增高架-2 (Autodesk Fusion 360 design; units mm, degrees)
part number: 2026-05-03-11-57-41-688
Autodesk Fusion 360 part; units mm, degrees
(part 1 of 12)
sketch "草图2" plane through (0, 0, 0) normal (0, 0, 1) x (1, 0, 0)
  line L0 (70.0002, -75) -> (70, 65) construction
  line L1 (60, 75) -> (-60, 75) construction
  line L2 (-70, 65) -> (-69.9998, -75) construction
  line L3 (-60, 75) -> (60, 75) construction
  line L4 (70, 85) -> (70, 165) construction
  line L5 (70, 165) -> (-70, 165) construction
  line L6 (-70, 165) -> (-70, 85) construction
  arc A0 (-70, 85) -> (-60, 75) centre (-60, 85) ccw construction
  arc A1 (-60, 75) -> (-70, 65) centre (-60, 65) ccw construction
  arc A2 (60, 75) -> (70, 85) centre (60, 85) ccw construction
  arc A3 (70, 65) -> (60, 75) centre (60, 65) ccw construction
  line L7 (-71.4998, -74.9987) -> (-68.4998, -74.9988)
  line L8 (68.5002, -74.9988) -> (71.5002, -74.9987)
  line L9 (68.5002, -74.9988) -> (68.5, 65)
  line L10 (71.5002, -74.9987) -> (71.5, 65)
  line L11 (60, 73.5) -> (-60, 73.5)
  line L12 (60, 76.5) -> (-60, 76.5)
  line L13 (-68.5, 65) -> (-68.4998, -74.9988)
  line L14 (-71.5, 65) -> (-71.4998, -74.9987)
  line L15 (68.5, 85.0003) -> (68.4999, 155)
  line L16 (71.5, 85.0232) -> (71.4999, 161.5)
  line L17 (59.9999, 163.5) -> (-60.0001, 163.5)
  line L18 (66.4999, 166.5) -> (-66.5001, 166.5)
  line L19 (-68.5001, 155) -> (-68.5, 85.0003)
  line L20 (-71.5001, 161.5) -> (-71.5, 85.0009)
  arc A4 (-68.5, 85.0003) -> (-60, 76.5) centre (-60, 85) ccw
  arc A5 (-60, 73.5) -> (-68.5, 65) centre (-60, 65) ccw
  arc A6 (60, 76.5) -> (68.5, 85.0003) centre (60, 85) ccw
  arc A7 (68.5, 65) -> (60, 73.5) centre (60, 65) ccw
  line L21 (-70, 65) -> (-70, 85) construction
  line L22 (70, 65) -> (70, 85) construction
  arc A8 (-71.5, 85.0009) -> (-71.5, 84.9991) centre (-60, 85) ccw
  arc A9 (71.5, 84.9769) -> (71.5, 85.0232) centre (60, 85) ccw
  line L23 (-71.5, 85.0009) -> (-71.5, 65)
  line L24 (71.5, 85.0232) -> (71.5, 65)
  arc A10 (-60.0001, 163.5) -> (-68.5001, 155) centre (-60.0001, 155) ccw
  arc A11 (-66.5001, 166.5) -> (-71.5001, 161.5) centre (-66.5001, 161.5) ccw
  arc A12 (68.4999, 155) -> (59.9999, 163.5) centre (59.9999, 155) ccw
  arc A13 (71.4999, 161.5) -> (66.4999, 166.5) centre (66.4999, 161.5) ccw
  dimension "d1" = 140
  dimension "d3" = 90
  dimension "d4" = 10
  dimension "d5" = 10
  dimension "d6" = 10
  dimension "d7" = 10
  dimension "d13" = 1.5
  dimension "d14" = 1.5
  dimension "d15" = 1.5
  dimension "d18" = 8.5
  dimension "d21" = 8.5
  dimension "d23" = 1.5
  dimension "d24" = 1.5
  dimension "d25" = 1.5
  dimension "d26" = 1.5
  dimension "d27" = 8.5
  dimension "d28" = 8.5
  dimension "d29" = 11.5
  dimension "d31" = 11.5
  dimension "d40" = 8.5
  dimension "d41" = 5
  dimension "d42" = 8.5
  dimension "d43" = 5
  constraint parallel L0 L2
  constraint perpendicular L3 L4
  constraint parallel L3 L5
  constraint parallel L4 L6
  constraint tangent L6 A0
  constraint tangent L3 A0
  constraint coincident L3 L1.end
  constraint tangent L3 A1
  constraint tangent L2 A1
  constraint tangent L4 A2
  constraint tangent L3 A2
  constraint tangent L1 A3
  constraint tangent L0 A3
  constraint coincident L7.start L14.end
  constraint coincident L7.end L13.end
  constraint coincident L8.start L9.start
  constraint coincident L8.end L10.start
  constraint coincident L9.end A7.start
  constraint coincident L11.start A7.end
  constraint coincident L11.end A5.start
  constraint coincident L12.start A6.start
  constraint coincident L12.end A4.end
  constraint coincident L13.start A5.end
  constraint coincident L15.start A6.end
  constraint coincident L19.end A4.start
  constraint parallel L0 L9
  constraint parallel L0 L10
  constraint parallel L1 L11
  constraint parallel L1 L12
  constraint parallel L2 L13
  constraint parallel L2 L14
  constraint parallel L0 L15
  constraint parallel L0 L16
  constraint parallel L5 L17
  constraint parallel L5 L18
  constraint parallel L2 L19
  constraint parallel L2 L20
  constraint concentric A0 A4
  constraint concentric A1 A5
  constraint concentric A2 A6
  constraint concentric A3 A7
  constraint coincident L2.start A1.end
  constraint coincident L6.end A0.start
  constraint coincident L0.end A3.start
  constraint coincident L4.start A2.end
  constraint coincident L16.start A9.end
  constraint coincident L20.end A8.start
  constraint concentric A0 A8
  constraint concentric A2 A9
  constraint coincident L23 A8.end
  constraint coincident L24 A9.start
  constraint tangent L17 A10
  constraint tangent L19 A10
  constraint tangent L20 A11
  constraint tangent L18 A11
  constraint tangent L17 A12
  constraint tangent L15 A12
  constraint tangent L16 A13
  constraint tangent L18 A13
  measures "d1" distance of L0 L2
  measures "d3" distance of L1 L5
  measures "d4" radius of A0
  measures "d5" radius of A1
  measures "d6" radius of A2
  measures "d7" radius of A3
  measures "d13" distance of L1 L11
  measures "d14" distance of L1 L12
  measures "d15" distance of L5 L17
  measures "d18" radius of A4
  measures "d21" radius of A6
  measures "d23" distance of L0 L9
  measures "d24" distance of L0 L10
  measures "d25" distance of L2 L13
  measures "d26" distance of L2 L14
  measures "d27" radius of A5
  measures "d28" radius of A7
  measures "d29" radius of A8
  measures "d31" radius of A9
  measures "d40" radius of A10
  measures "d41" radius of A11
  measures "d42" radius of A12
  measures "d43" radius of A13
extrude "拉伸1" add sketch "草图2" along normal blind 250 contours L7 L13 L14 A5 A8 L23 | L12 L19 A4 A8 | L8 L9 L10 L11 L12 L15 L16 L17 L18 L19 L20 A6 A7 A8 A9 L24 A10 A11 A12 A13 picked at (-59.4355, 74.5418)
sketch "草图18" plane through (0, 166.5, 0) normal (0, 1, 0) x (-1, 0, 0)
  line L0 (-66.4999, 0) -> (66.5001, 0)
  line L1 (66.5001, 0) -> (66.5001, 250)
  line L2 (66.5001, 250) -> (-66.4999, 250)
  line L3 (-66.4999, 250) -> (-66.4999, 0)
  line L4 (-56.4999, 15) -> (-60.83, 12.5)
  line L5 (-60.83, 12.5) -> (-60.83, 7.5)
  line L6 (-60.83, 7.5) -> (-56.4999, 5)
  line L7 (-56.4999, 5) -> (-52.1698, 7.5)
  line L8 (-52.1698, 7.5) -> (-52.1698, 12.5)
  line L9 (-52.1698, 12.5) -> (-56.4999, 15)
  line L10 (-45.8396, 15) -> (-50.1698, 12.5)
  line L11 (-50.1698, 12.5) -> (-50.1698, 7.5)
  line L12 (-50.1698, 7.5) -> (-45.8396, 5)
  line L13 (-45.8396, 5) -> (-41.5095, 7.5)
  line L14 (-41.5095, 7.5) -> (-41.5095, 12.5)
  line L15 (-41.5095, 12.5) -> (-45.8396, 15)
  line L16 (-35.1794, 15) -> (-39.5095, 12.5)
  line L17 (-39.5095, 12.5) -> (-39.5095, 7.5)
  line L18 (-39.5095, 7.5) -> (-35.1794, 5)
  line L19 (-35.1794, 5) -> (-30.8493, 7.5)
  line L20 (-30.8493, 7.5) -> (-30.8493, 12.5)
  line L21 (-30.8493, 12.5) -> (-35.1794, 15)
  line L22 (-24.5191, 15) -> (-28.8493, 12.5)
  line L23 (-28.8493, 12.5) -> (-28.8493, 7.5)
  line L24 (-28.8493, 7.5) -> (-24.5191, 5)
  line L25 (-24.5191, 5) -> (-20.189, 7.5)
  line L26 (-20.189, 7.5) -> (-20.189, 12.5)
  line L27 (-20.189, 12.5) -> (-24.5191, 15)
  line L28 (-13.8589, 15) -> (-18.189, 12.5)
  line L29 (-18.189, 12.5) -> (-18.189, 7.5)
  line L30 (-18.189, 7.5) -> (-13.8589, 5)
  line L31 (-13.8589, 5) -> (-9.5287, 7.5)
  line L32 (-9.5287, 7.5) -> (-9.5287, 12.5)
  line L33 (-9.5287, 12.5) -> (-13.8589, 15)
  line L34 (-3.1986, 15) -> (-7.5287, 12.5)
  line L35 (-7.5287, 12.5) -> (-7.5287, 7.5)
  line L36 (-7.5287, 7.5) -> (-3.1986, 5)
  line L37 (-3.1986, 5) -> (1.1315, 7.5)
  line L38 (1.1315, 7.5) -> (1.1315, 12.5)
  line L39 (1.1315, 12.5) -> (-3.1986, 15)
  line L40 (7.4616, 15) -> (3.1315, 12.5)
  line L41 (3.1315, 12.5) -> (3.1315, 7.5)
  line L42 (3.1315, 7.5) -> (7.4616, 5)
  line L43 (7.4616, 5) -> (11.7918, 7.5)
  line L44 (11.7918, 7.5) -> (11.7918, 12.5)
  line L45 (11.7918, 12.5) -> (7.4616, 15)
  line L46 (18.1219, 15) -> (13.7918, 12.5)
  line L47 (13.7918, 12.5) -> (13.7918, 7.5)
  line L48 (13.7918, 7.5) -> (18.1219, 5)
  line L49 (18.1219, 5) -> (22.452, 7.5)
  line L50 (22.452, 7.5) -> (22.452, 12.5)
  line L51 (22.452, 12.5) -> (18.1219, 15)
  line L52 (28.7821, 15) -> (24.452, 12.5)
  line L53 (24.452, 12.5) -> (24.452, 7.5)
  line L54 (24.452, 7.5) -> (28.7821, 5)
  line L55 (28.7821, 5) -> (33.1123, 7.5)
  line L56 (33.1123, 7.5) -> (33.1123, 12.5)
  line L57 (33.1123, 12.5) -> (28.7821, 15)
  line L58 (39.4424, 15) -> (35.1123, 12.5)
  line L59 (35.1123, 12.5) -> (35.1123, 7.5)
  line L60 (35.1123, 7.5) -> (39.4424, 5)
  line L61 (39.4424, 5) -> (43.7725, 7.5)
  line L62 (43.7725, 7.5) -> (43.7725, 12.5)
  line L63 (43.7725, 12.5) -> (39.4424, 15)
  line L64 (50.1027, 15) -> (45.7725, 12.5)
  line L65 (45.7725, 12.5) -> (45.7725, 7.5)
  line L66 (45.7725, 7.5) -> (50.1027, 5)
  line L67 (50.1027, 5) -> (54.4328, 7.5)
  line L68 (54.4328, 7.5) -> (54.4328, 12.5)
  line L69 (54.4328, 12.5) -> (50.1027, 15)
  line L70 (-51.1698, 24.2321) -> (-55.4999, 21.7321)
  line L71 (-55.4999, 21.7321) -> (-55.4999, 16.7321)
  line L72 (-55.4999, 16.7321) -> (-51.1698, 14.2321)
  line L73 (-51.1698, 14.2321) -> (-46.8396, 16.7321)
  line L74 (-46.8396, 16.7321) -> (-46.8396, 21.7321)
  line L75 (-46.8396, 21.7321) -> (-51.1698, 24.2321)
  line L76 (-40.5095, 24.2321) -> (-44.8396, 21.7321)
  line L77 (-44.8396, 21.7321) -> (-44.8396, 16.7321)
  line L78 (-44.8396, 16.7321) -> (-40.5095, 14.2321)
  line L79 (-40.5095, 14.2321) -> (-36.1794, 16.7321)
  line L80 (-36.1794, 16.7321) -> (-36.1794, 21.7321)
  line L81 (-36.1794, 21.7321) -> (-40.5095, 24.2321)
  line L82 (-29.8493, 24.2321) -> (-34.1794, 21.7321)
  line L83 (-34.1794, 21.7321) -> (-34.1794, 16.7321)
  line L84 (-34.1794, 16.7321) -> (-29.8493, 14.2321)
  line L85 (-29.8493, 14.2321) -> (-25.5191, 16.7321)
  line L86 (-25.5191, 16.7321) -> (-25.5191, 21.7321)
  line L87 (-25.5191, 21.7321) -> (-29.8493, 24.2321)
  line L88 (-19.189, 24.2321) -> (-23.5191, 21.7321)
  line L89 (-23.5191, 21.7321) -> (-23.5191, 16.7321)
  line L90 (-23.5191, 16.7321) -> (-19.189, 14.2321)
  line L91 (-19.189, 14.2321) -> (-14.8589, 16.7321)
  line L92 (-14.8589, 16.7321) -> (-14.8589, 21.7321)
  line L93 (-14.8589, 21.7321) -> (-19.189, 24.2321)
  line L94 (-8.5287, 24.2321) -> (-12.8589, 21.7321)
  line L95 (-12.8589, 21.7321) -> (-12.8589, 16.7321)
  line L96 (-12.8589, 16.7321) -> (-8.5287, 14.2321)
  line L97 (-8.5287, 14.2321) -> (-4.1986, 16.7321)
  line L98 (-4.1986, 16.7321) -> (-4.1986, 21.7321)
  line L99 (-4.1986, 21.7321) -> (-8.5287, 24.2321)
  line L100 (2.1315, 24.2321) -> (-2.1986, 21.7321)
  line L101 (-2.1986, 21.7321) -> (-2.1986, 16.7321)
  line L102 (-2.1986, 16.7321) -> (2.1315, 14.2321)
  line L103 (2.1315, 14.2321) -> (6.4616, 16.7321)
  line L104 (6.4616, 16.7321) -> (6.4616, 21.7321)
  line L105 (6.4616, 21.7321) -> (2.1315, 24.2321)
  line L106 (12.7918, 24.2321) -> (8.4616, 21.7321)
  line L107 (8.4616, 21.7321) -> (8.4616, 16.7321)
  line L108 (8.4616, 16.7321) -> (12.7918, 14.2321)
  line L109 (12.7918, 14.2321) -> (17.1219, 16.7321)
  line L110 (17.1219, 16.7321) -> (17.1219, 21.7321)
  line L111 (17.1219, 21.7321) -> (12.7918, 24.2321)
  line L112 (23.452, 24.2321) -> (19.1219, 21.7321)
  line L113 (19.1219, 21.7321) -> (19.1219, 16.7321)
  line L114 (19.1219, 16.7321) -> (23.452, 14.2321)
  line L115 (23.452, 14.2321) -> (27.7821, 16.7321)
  line L116 (27.7821, 16.7321) -> (27.7821, 21.7321)
  line L117 (27.7821, 21.7321) -> (23.452, 24.2321)
  line L118 (34.1123, 24.2321) -> (29.7821, 21.7321)
  line L119 (29.7821, 21.7321) -> (29.7821, 16.7321)
  line L120 (29.7821, 16.7321) -> (34.1123, 14.2321)
  line L121 (34.1123, 14.2321) -> (38.4424, 16.7321)
  line L122 (38.4424, 16.7321) -> (38.4424, 21.7321)
  line L123 (38.4424, 21.7321) -> (34.1123, 24.2321)
  line L124 (44.7725, 24.2321) -> (40.4424, 21.7321)
  line L125 (40.4424, 21.7321) -> (40.4424, 16.7321)
  line L126 (40.4424, 16.7321) -> (44.7725, 14.2321)
  line L127 (44.7725, 14.2321) -> (49.1027, 16.7321)
  line L128 (49.1027, 16.7321) -> (49.1027, 21.7321)
  line L129 (49.1027, 21.7321) -> (44.7725, 24.2321)
  line L130 (55.4328, 24.2321) -> (51.1027, 21.7321)
  line L131 (51.1027, 21.7321) -> (51.1027, 16.7321)
  line L132 (51.1027, 16.7321) -> (55.4328, 14.2321)
  line L133 (55.4328, 14.2321) -> (59.7629, 16.7321)
  line L134 (59.7629, 16.7321) -> (59.7629, 21.7321)
  line L135 (59.7629, 21.7321) -> (55.4328, 24.2321)
  line L136 (-56.4999, 33.4641) -> (-60.83, 30.9641)
  line L137 (-60.83, 30.9641) -> (-60.83, 25.9641)
  line L138 (-60.83, 25.9641) -> (-56.4999, 23.4641)
  line L139 (-56.4999, 23.4641) -> (-52.1698, 25.9641)
  line L140 (-52.1698, 25.9641) -> (-52.1698, 30.9641)
  line L141 (-52.1698, 30.9641) -> (-56.4999, 33.4641)
  line L142 (-45.8396, 33.4641) -> (-50.1698, 30.9641)
  line L143 (-50.1698, 30.9641) -> (-50.1698, 25.9641)
  line L144 (-50.1698, 25.9641) -> (-45.8396, 23.4641)
  line L145 (-45.8396, 23.4641) -> (-41.5095, 25.9641)
  line L146 (-41.5095, 25.9641) -> (-41.5095, 30.9641)
  line L147 (-41.5095, 30.9641) -> (-45.8396, 33.4641)
  line L148 (-35.1794, 33.4641) -> (-39.5095, 30.9641)
  line L149 (-39.5095, 30.9641) -> (-39.5095, 25.9641)
  line L150 (-39.5095, 25.9641) -> (-35.1794, 23.4641)
  line L151 (-35.1794, 23.4641) -> (-30.8493, 25.9641)
  line L152 (-30.8493, 25.9641) -> (-30.8493, 30.9641)
  line L153 (-30.8493, 30.9641) -> (-35.1794, 33.4641)
  line L154 (-24.5191, 33.4641) -> (-28.8493, 30.9641)
  line L155 (-28.8493, 30.9641) -> (-28.8493, 25.9641)
  line L156 (-28.8493, 25.9641) -> (-24.5191, 23.4641)
  line L157 (-24.5191, 23.4641) -> (-20.189, 25.9641)
  line L158 (-20.189, 25.9641) -> (-20.189, 30.9641)
  line L159 (-20.189, 30.9641) -> (-24.5191, 33.4641)
  line L160 (-13.8589, 33.4641) -> (-18.189, 30.9641)
  line L161 (-18.189, 30.9641) -> (-18.189, 25.9641)
  line L162 (-18.189, 25.9641) -> (-13.8589, 23.4641)
  line L163 (-13.8589, 23.4641) -> (-9.5287, 25.9641)
  line L164 (-9.5287, 25.9641) -> (-9.5287, 30.9641)
  line L165 (-9.5287, 30.9641) -> (-13.8589, 33.4641)
  line L166 (-3.1986, 33.4641) -> (-7.5287, 30.9641)
  line L167 (-7.5287, 30.9641) -> (-7.5287, 25.9641)
  line L168 (-7.5287, 25.9641) -> (-3.1986, 23.4641)
  line L169 (-3.1986, 23.4641) -> (1.1315, 25.9641)
  line L170 (1.1315, 25.9641) -> (1.1315, 30.9641)
  line L171 (1.1315, 30.9641) -> (-3.1986, 33.4641)
  line L172 (7.4616, 33.4641) -> (3.1315, 30.9641)
  line L173 (3.1315, 30.9641) -> (3.1315, 25.9641)
  line L174 (3.1315, 25.9641) -> (7.4616, 23.4641)
  line L175 (7.4616, 23.4641) -> (11.7918, 25.9641)
  line L176 (11.7918, 25.9641) -> (11.7918, 30.9641)
  line L177 (11.7918, 30.9641) -> (7.4616, 33.4641)
  line L178 (18.1219, 33.4641) -> (13.7918, 30.9641)
  line L179 (13.7918, 30.9641) -> (13.7918, 25.9641)
  line L180 (13.7918, 25.9641) -> (18.1219, 23.4641)
  line L181 (18.1219, 23.4641) -> (22.452, 25.9641)
  line L182 (22.452, 25.9641) -> (22.452, 30.9641)
  line L183 (22.452, 30.9641) -> (18.1219, 33.4641)
  line L184 (28.7821, 33.4641) -> (24.452, 30.9641)
  line L185 (24.452, 30.9641) -> (24.452, 25.9641)
  line L186 (24.452, 25.9641) -> (28.7821, 23.4641)
  line L187 (28.7821, 23.4641) -> (33.1123, 25.9641)
  line L188 (33.1123, 25.9641) -> (33.1123, 30.9641)
  line L189 (33.1123, 30.9641) -> (28.7821, 33.4641)
  line L190 (39.4424, 33.4641) -> (35.1123, 30.9641)
  line L191 (35.1123, 30.9641) -> (35.1123, 25.9641)
  line L192 (35.1123, 25.9641) -> (39.4424, 23.4641)
  line L193 (39.4424, 23.4641) -> (43.7725, 25.9641)
  line L194 (43.7725, 25.9641) -> (43.7725, 30.9641)
  line L195 (43.7725, 30.9641) -> (39.4424, 33.4641)
  line L196 (50.1027, 33.4641) -> (45.7725, 30.9641)
  line L197 (45.7725, 30.9641) -> (45.7725, 25.9641)
  line L198 (45.7725, 25.9641) -> (50.1027, 23.4641)
  line L199 (50.1027, 23.4641) -> (54.4328, 25.9641)
  line L200 (54.4328, 25.9641) -> (54.4328, 30.9641)
  line L201 (54.4328, 30.9641) -> (50.1027, 33.4641)
  line L202 (-51.1698, 42.6962) -> (-55.4999, 40.1962)
  line L203 (-55.4999, 40.1962) -> (-55.4999, 35.1962)
  line L204 (-55.4999, 35.1962) -> (-51.1698, 32.6962)
  line L205 (-51.1698, 32.6962) -> (-46.8396, 35.1962)
  line L206 (-46.8396, 35.1962) -> (-46.8396, 40.1962)
  line L207 (-46.8396, 40.1962) -> (-51.1698, 42.6962)
  line L208 (-40.5095, 42.6962) -> (-44.8396, 40.1962)
  line L209 (-44.8396, 40.1962) -> (-44.8396, 35.1962)
  line L210 (-44.8396, 35.1962) -> (-40.5095, 32.6962)
  line L211 (-40.5095, 32.6962) -> (-36.1794, 35.1962)
  line L212 (-36.1794, 35.1962) -> (-36.1794, 40.1962)
  line L213 (-36.1794, 40.1962) -> (-40.5095, 42.6962)
  line L214 (-29.8493, 42.6962) -> (-34.1794, 40.1962)
  line L215 (-34.1794, 40.1962) -> (-34.1794, 35.1962)
  line L216 (-34.1794, 35.1962) -> (-29.8493, 32.6962)
  line L217 (-29.8493, 32.6962) -> (-25.5191, 35.1962)
  line L218 (-25.5191, 35.1962) -> (-25.5191, 40.1962)
  line L219 (-25.5191, 40.1962) -> (-29.8493, 42.6962)
  line L220 (-19.189, 42.6962) -> (-23.5191, 40.1962)
  line L221 (-23.5191, 40.1962) -> (-23.5191, 35.1962)
  line L222 (-23.5191, 35.1962) -> (-19.189, 32.6962)
  line L223 (-19.189, 32.6962) -> (-14.8589, 35.1962)
  line L224 (-14.8589, 35.1962) -> (-14.8589, 40.1962)
  line L225 (-14.8589, 40.1962) -> (-19.189, 42.6962)
  line L226 (-8.5287, 42.6962) -> (-12.8589, 40.1962)
  line L227 (-12.8589, 40.1962) -> (-12.8589, 35.1962)
  line L228 (-12.8589, 35.1962) -> (-8.5287, 32.6962)
  line L229 (-8.5287, 32.6962) -> (-4.1986, 35.1962)
  line L230 (-4.1986, 35.1962) -> (-4.1986, 40.1962)
  line L231 (-4.1986, 40.1962) -> (-8.5287, 42.6962)
  line L232 (2.1315, 42.6962) -> (-2.1986, 40.1962)
  line L233 (-2.1986, 40.1962) -> (-2.1986, 35.1962)
  line L234 (-2.1986, 35.1962) -> (2.1315, 32.6962)
  line L235 (2.1315, 32.6962) -> (6.4616, 35.1962)
  line L236 (6.4616, 35.1962) -> (6.4616, 40.1962)
  line L237 (6.4616, 40.1962) -> (2.1315, 42.6962)
  line L238 (12.7918, 42.6962) -> (8.4616, 40.1962)
  line L239 (8.4616, 40.1962) -> (8.4616, 35.1962)
  line L240 (8.4616, 35.1962) -> (12.7918, 32.6962)
  line L241 (12.7918, 32.6962) -> (17.1219, 35.1962)
  line L242 (17.1219, 35.1962) -> (17.1219, 40.1962)
  line L243 (17.1219, 40.1962) -> (12.7918, 42.6962)
  line L244 (23.452, 42.6962) -> (19.1219, 40.1962)
  line L245 (19.1219, 40.1962) -> (19.1219, 35.1962)
  line L246 (19.1219, 35.1962) -> (23.452, 32.6962)
  line L247 (23.452, 32.6962) -> (27.7821, 35.1962)
  line L248 (27.7821, 35.1962) -> (27.7821, 40.1962)
  line L249 (27.7821, 40.1962) -> (23.452, 42.6962)
  line L250 (34.1123, 42.6962) -> (29.7821, 40.1962)
  line L251 (29.7821, 40.1962) -> (29.7821, 35.1962)
  line L252 (29.7821, 35.1962) -> (34.1123, 32.6962)
  line L253 (34.1123, 32.6962) -> (38.4424, 35.1962)
  line L254 (38.4424, 35.1962) -> (38.4424, 40.1962)
  line L255 (38.4424, 40.1962) -> (34.1123, 42.6962)
  line L256 (44.7725, 42.6962) -> (40.4424, 40.1962)
  line L257 (40.4424, 40.1962) -> (40.4424, 35.1962)
  line L258 (40.4424, 35.1962) -> (44.7725, 32.6962)
  line L259 (44.7725, 32.6962) -> (49.1027, 35.1962)
  line L260 (49.1027, 35.1962) -> (49.1027, 40.1962)
  line L261 (49.1027, 40.1962) -> (44.7725, 42.6962)
  line L262 (55.4328, 42.6962) -> (51.1027, 40.1962)
  line L263 (51.1027, 40.1962) -> (51.1027, 35.1962)
  line L264 (51.1027, 35.1962) -> (55.4328, 32.6962)
  line L265 (55.4328, 32.6962) -> (59.7629, 35.1962)
  line L266 (59.7629, 35.1962) -> (59.7629, 40.1962)
  line L267 (59.7629, 40.1962) -> (55.4328, 42.6962)
  line L268 (-56.4999, 51.9282) -> (-60.83, 49.4282)
  line L269 (-60.83, 49.4282) -> (-60.83, 44.4282)
  line L270 (-60.83, 44.4282) -> (-56.4999, 41.9282)
  line L271 (-56.4999, 41.9282) -> (-52.1698, 44.4282)
  line L272 (-52.1698, 44.4282) -> (-52.1698, 49.4282)
  line L273 (-52.1698, 49.4282) -> (-56.4999, 51.9282)
  line L274 (-45.8396, 51.9282) -> (-50.1698, 49.4282)
  line L275 (-50.1698, 49.4282) -> (-50.1698, 44.4282)
  line L276 (-50.1698, 44.4282) -> (-45.8396, 41.9282)
  line L277 (-45.8396, 41.9282) -> (-41.5095, 44.4282)
  line L278 (-41.5095, 44.4282) -> (-41.5095, 49.4282)
  line L279 (-41.5095, 49.4282) -> (-45.8396, 51.9282)
  line L280 (-35.1794, 51.9282) -> (-39.5095, 49.4282)
  line L281 (-39.5095, 49.4282) -> (-39.5095, 44.4282)
  line L282 (-39.5095, 44.4282) -> (-35.1794, 41.9282)
  line L283 (-35.1794, 41.9282) -> (-30.8493, 44.4282)
  line L284 (-30.8493, 44.4282) -> (-30.8493, 49.4282)
  line L285 (-30.8493, 49.4282) -> (-35.1794, 51.9282)
  line L286 (-24.5191, 51.9282) -> (-28.8493, 49.4282)
  line L287 (-28.8493, 49.4282) -> (-28.8493, 44.4282)
  line L288 (-28.8493, 44.4282) -> (-24.5191, 41.9282)
  line L289 (-24.5191, 41.9282) -> (-20.189, 44.4282)
  line L290 (-20.189, 44.4282) -> (-20.189, 49.4282)
  line L291 (-20.189, 49.4282) -> (-24.5191, 51.9282)
  line L292 (-13.8589, 51.9282) -> (-18.189, 49.4282)
  line L293 (-18.189, 49.4282) -> (-18.189, 44.4282)
  line L294 (-18.189, 44.4282) -> (-13.8589, 41.9282)
  line L295 (-13.8589, 41.9282) -> (-9.5287, 44.4282)
  line L296 (-9.5287, 44.4282) -> (-9.5287, 49.4282)
  line L297 (-9.5287, 49.4282) -> (-13.8589, 51.9282)
  line L298 (-3.1986, 51.9282) -> (-7.5287, 49.4282)
  line L299 (-7.5287, 49.4282) -> (-7.5287, 44.4282)
  line L300 (-7.5287, 44.4282) -> (-3.1986, 41.9282)
  line L301 (-3.1986, 41.9282) -> (1.1315, 44.4282)
  line L302 (1.1315, 44.4282) -> (1.1315, 49.4282)
  line L303 (1.1315, 49.4282) -> (-3.1986, 51.9282)
  line L304 (7.4616, 51.9282) -> (3.1315, 49.4282)
  line L305 (3.1315, 49.4282) -> (3.1315, 44.4282)
  line L306 (3.1315, 44.4282) -> (7.4616, 41.9282)
  line L307 (7.4616, 41.9282) -> (11.7918, 44.4282)
  line L308 (11.7918, 44.4282) -> (11.7918, 49.4282)
  line L309 (11.7918, 49.4282) -> (7.4616, 51.9282)
  line L310 (18.1219, 51.9282) -> (13.7918, 49.4282)
  line L311 (13.7918, 49.4282) -> (13.7918, 44.4282)
  line L312 (13.7918, 44.4282) -> (18.1219, 41.9282)
  line L313 (18.1219, 41.9282) -> (22.452, 44.4282)
  line L314 (22.452, 44.4282) -> (22.452, 49.4282)
  line L315 (22.452, 49.4282) -> (18.1219, 51.9282)
  line L316 (28.7821, 51.9282) -> (24.452, 49.4282)
  line L317 (24.452, 49.4282) -> (24.452, 44.4282)
  line L318 (24.452, 44.4282) -> (28.7821, 41.9282)
  line L319 (28.7821, 41.9282) -> (33.1123, 44.4282)
  line L320 (33.1123, 44.4282) -> (33.1123, 49.4282)
  line L321 (33.1123, 49.4282) -> (28.7821, 51.9282)
  line L322 (39.4424, 51.9282) -> (35.1123, 49.4282)
  line L323 (35.1123, 49.4282) -> (35.1123, 44.4282)
  line L324 (35.1123, 44.4282) -> (39.4424, 41.9282)
  line L325 (39.4424, 41.9282) -> (43.7725, 44.4282)
  line L326 (43.7725, 44.4282) -> (43.7725, 49.4282)
  line L327 (43.7725, 49.4282) -> (39.4424, 51.9282)
  line L328 (50.1027, 51.9282) -> (45.7725, 49.4282)
  line L329 (45.7725, 49.4282) -> (45.7725, 44.4282)
  line L330 (45.7725, 44.4282) -> (50.1027, 41.9282)
  line L331 (50.1027, 41.9282) -> (54.4328, 44.4282)
  line L332 (54.4328, 44.4282) -> (54.4328, 49.4282)
  line L333 (54.4328, 49.4282) -> (50.1027, 51.9282)
  line L334 (-51.1698, 61.1603) -> (-55.4999, 58.6603)
  line L335 (-55.4999, 58.6603) -> (-55.4999, 53.6603)
  line L336 (-55.4999, 53.6603) -> (-51.1698, 51.1603)
  line L337 (-51.1698, 51.1603) -> (-46.8396, 53.6603)
  line L338 (-46.8396, 53.6603) -> (-46.8396, 58.6603)
  line L339 (-46.8396, 58.6603) -> (-51.1698, 61.1603)
  line L340 (-40.5095, 61.1603) -> (-44.8396, 58.6603)
  line L341 (-44.8396, 58.6603) -> (-44.8396, 53.6603)
  line L342 (-44.8396, 53.6603) -> (-40.5095, 51.1603)
  line L343 (-40.5095, 51.1603) -> (-36.1794, 53.6603)
  line L344 (-36.1794, 53.6603) -> (-36.1794, 58.6603)
  line L345 (-36.1794, 58.6603) -> (-40.5095, 61.1603)
  line L346 (-29.8493, 61.1603) -> (-34.1794, 58.6603)
  line L347 (-34.1794, 58.6603) -> (-34.1794, 53.6603)
  line L348 (-34.1794, 53.6603) -> (-29.8493, 51.1603)
  line L349 (-29.8493, 51.1603) -> (-25.5191, 53.6603)
  line L350 (-25.5191, 53.6603) -> (-25.5191, 58.6603)
  line L351 (-25.5191, 58.6603) -> (-29.8493, 61.1603)
  line L352 (-19.189, 61.1603) -> (-23.5191, 58.6603)
  line L353 (-23.5191, 58.6603) -> (-23.5191, 53.6603)
  line L354 (-23.5191, 53.6603) -> (-19.189, 51.1603)
  line L355 (-19.189, 51.1603) -> (-14.8589, 53.6603)
  line L356 (-14.8589, 53.6603) -> (-14.8589, 58.6603)
  line L357 (-14.8589, 58.6603) -> (-19.189, 61.1603)
  line L358 (-8.5287, 61.1603) -> (-12.8589, 58.6603)
  line L359 (-12.8589, 58.6603) -> (-12.8589, 53.6603)
  line L360 (-12.8589, 53.6603) -> (-8.5287, 51.1603)
  line L361 (-8.5287, 51.1603) -> (-4.1986, 53.6603)
  line L362 (-4.1986, 53.6603) -> (-4.1986, 58.6603)
  line L363 (-4.1986, 58.6603) -> (-8.5287, 61.1603)
  line L364 (2.1315, 61.1603) -> (-2.1986, 58.6603)
  line L365 (-2.1986, 58.6603) -> (-2.1986, 53.6603)
  line L366 (-2.1986, 53.6603) -> (2.1315, 51.1603)
  line L367 (2.1315, 51.1603) -> (6.4616, 53.6603)
  line L368 (6.4616, 53.6603) -> (6.4616, 58.6603)
  line L369 (6.4616, 58.6603) -> (2.1315, 61.1603)
  line L370 (12.7918, 61.1603) -> (8.4616, 58.6603)
  line L371 (8.4616, 58.6603) -> (8.4616, 53.6603)
  line L372 (8.4616, 53.6603) -> (12.7918, 51.1603)
  line L373 (12.7918, 51.1603) -> (17.1219, 53.6603)
  line L374 (17.1219, 53.6603) -> (17.1219, 58.6603)
  line L375 (17.1219, 58.6603) -> (12.7918, 61.1603)
  line L376 (23.452, 61.1603) -> (19.1219, 58.6603)
  line L377 (19.1219, 58.6603) -> (19.1219, 53.6603)
  line L378 (19.1219, 53.6603) -> (23.452, 51.1603)
  line L379 (23.452, 51.1603) -> (27.7821, 53.6603)
  line L380 (27.7821, 53.6603) -> (27.7821, 58.6603)
  line L381 (27.7821, 58.6603) -> (23.452, 61.1603)
  line L382 (34.1123, 61.1603) -> (29.7821, 58.6603)
  line L383 (29.7821, 58.6603) -> (29.7821, 53.6603)
  line L384 (29.7821, 53.6603) -> (34.1123, 51.1603)
  line L385 (34.1123, 51.1603) -> (38.4424, 53.6603)
  line L386 (38.4424, 53.6603) -> (38.4424, 58.6603)
  line L387 (38.4424, 58.6603) -> (34.1123, 61.1603)
  line L388 (44.7725, 61.1603) -> (40.4424, 58.6603)
  line L389 (40.4424, 58.6603) -> (40.4424, 53.6603)
  line L390 (40.4424, 53.6603) -> (44.7725, 51.1603)
  line L391 (44.7725, 51.1603) -> (49.1027, 53.6603)
  line L392 (49.1027, 53.6603) -> (49.1027, 58.6603)
  line L393 (49.1027, 58.6603) -> (44.7725, 61.1603)
  line L394 (55.4328, 61.1603) -> (51.1027, 58.6603)
  line L395 (51.1027, 58.6603) -> (51.1027, 53.6603)
  line L396 (51.1027, 53.6603) -> (55.4328, 51.1603)
  line L397 (55.4328, 51.1603) -> (59.7629, 53.6603)
  line L398 (59.7629, 53.6603) -> (59.7629, 58.6603)
  line L399 (59.7629, 58.6603) -> (55.4328, 61.1603)
  line L400 (-56.4999, 70.3923) -> (-60.83, 67.8923)
  line L401 (-60.83, 67.8923) -> (-60.83, 62.8923)
  line L402 (-60.83, 62.8923) -> (-56.4999, 60.3923)
  line L403 (-56.4999, 60.3923) -> (-52.1698, 62.8923)
  line L404 (-52.1698, 62.8923) -> (-52.1698, 67.8923)
  line L405 (-52.1698, 67.8923) -> (-56.4999, 70.3923)
  line L406 (-45.8396, 70.3923) -> (-50.1698, 67.8923)
  line L407 (-50.1698, 67.8923) -> (-50.1698, 62.8923)
  line L408 (-50.1698, 62.8923) -> (-45.8396, 60.3923)
  line L409 (-45.8396, 60.3923) -> (-41.5095, 62.8923)
  line L410 (-41.5095, 62.8923) -> (-41.5095, 67.8923)
  line L411 (-41.5095, 67.8923) -> (-45.8396, 70.3923)
  line L412 (-35.1794, 70.3923) -> (-39.5095, 67.8923)
  line L413 (-39.5095, 67.8923) -> (-39.5095, 62.8923)
  line L414 (-39.5095, 62.8923) -> (-35.1794, 60.3923)
  line L415 (-35.1794, 60.3923) -> (-30.8493, 62.8923)
  line L416 (-30.8493, 62.8923) -> (-30.8493, 67.8923)
  line L417 (-30.8493, 67.8923) -> (-35.1794, 70.3923)
  line L418 (-24.5191, 70.3923) -> (-28.8493, 67.8923)
  line L419 (-28.8493, 67.8923) -> (-28.8493, 62.8923)
  line L420 (-28.8493, 62.8923) -> (-24.5191, 60.3923)
  line L421 (-24.5191, 60.3923) -> (-20.189, 62.8923)
  line L422 (-20.189, 62.8923) -> (-20.189, 67.8923)
  line L423 (-20.189, 67.8923) -> (-24.5191, 70.3923)
  line L424 (-13.8589, 70.3923) -> (-18.189, 67.8923)
  line L425 (-18.189, 67.8923) -> (-18.189, 62.8923)
  line L426 (-18.189, 62.8923) -> (-13.8589, 60.3923)
  line L427 (-13.8589, 60.3923) -> (-9.5287, 62.8923)
  line L428 (-9.5287, 62.8923) -> (-9.5287, 67.8923)
  line L429 (-9.5287, 67.8923) -> (-13.8589, 70.3923)
  line L430 (-3.1986, 70.3923) -> (-7.5287, 67.8923)
  line L431 (-7.5287, 67.8923) -> (-7.5287, 62.8923)
  line L432 (-7.5287, 62.8923) -> (-3.1986, 60.3923)
  line L433 (-3.1986, 60.3923) -> (1.1315, 62.8923)
  line L434 (1.1315, 62.8923) -> (1.1315, 67.8923)
  line L435 (1.1315, 67.8923) -> (-3.1986, 70.3923)
  line L436 (7.4616, 70.3923) -> (3.1315, 67.8923)
  line L437 (3.1315, 67.8923) -> (3.1315, 62.8923)
  line L438 (3.1315, 62.8923) -> (7.4616, 60.3923)
  line L439 (7.4616, 60.3923) -> (11.7918, 62.8923)
  line L440 (11.7918, 62.8923) -> (11.7918, 67.8923)
  line L441 (11.7918, 67.8923) -> (7.4616, 70.3923)
  line L442 (18.1219, 70.3923) -> (13.7918, 67.8923)
  line L443 (13.7918, 67.8923) -> (13.7918, 62.8923)
  line L444 (13.7918, 62.8923) -> (18.1219, 60.3923)
  line L445 (18.1219, 60.3923) -> (22.452, 62.8923)
  line L446 (22.452, 62.8923) -> (22.452, 67.8923)
  line L447 (22.452, 67.8923) -> (18.1219, 70.3923)
  line L448 (28.7821, 70.3923) -> (24.452, 67.8923)
  line L449 (24.452, 67.8923) -> (24.452, 62.8923)
  line L450 (24.452, 62.8923) -> (28.7821, 60.3923)
  line L451 (28.7821, 60.3923) -> (33.1123, 62.8923)
  line L452 (33.1123, 62.8923) -> (33.1123, 67.8923)
  line L453 (33.1123, 67.8923) -> (28.7821, 70.3923)
  line L454 (39.4424, 70.3923) -> (35.1123, 67.8923)
  line L455 (35.1123, 67.8923) -> (35.1123, 62.8923)
  line L456 (35.1123, 62.8923) -> (39.4424, 60.3923)
  line L457 (39.4424, 60.3923) -> (43.7725, 62.8923)
  line L458 (43.7725, 62.8923) -> (43.7725, 67.8923)
  line L459 (43.7725, 67.8923) -> (39.4424, 70.3923)
  line L460 (50.1027, 70.3923) -> (45.7725, 67.8923)
  line L461 (45.7725, 67.8923) -> (45.7725, 62.8923)
  line L462 (45.7725, 62.8923) -> (50.1027, 60.3923)
  line L463 (50.1027, 60.3923) -> (54.4328, 62.8923)
  line L464 (54.4328, 62.8923) -> (54.4328, 67.8923)
  line L465 (54.4328, 67.8923) -> (50.1027, 70.3923)
  line L466 (-51.1698, 79.6244) -> (-55.4999, 77.1244)
  line L467 (-55.4999, 77.1244) -> (-55.4999, 72.1244)
  line L468 (-55.4999, 72.1244) -> (-51.1698, 69.6244)
  line L469 (-51.1698, 69.6244) -> (-46.8396, 72.1244)
  line L470 (-46.8396, 72.1244) -> (-46.8396, 77.1244)
  line L471 (-46.8396, 77.1244) -> (-51.1698, 79.6244)
  line L472 (-40.5095, 79.6244) -> (-44.8396, 77.1244)
  line L473 (-44.8396, 77.1244) -> (-44.8396, 72.1244)
  line L474 (-44.8396, 72.1244) -> (-40.5095, 69.6244)
  line L475 (-40.5095, 69.6244) -> (-36.1794, 72.1244)
  line L476 (-36.1794, 72.1244) -> (-36.1794, 77.1244)
  line L477 (-36.1794, 77.1244) -> (-40.5095, 79.6244)
  line L478 (-29.8493, 79.6244) -> (-34.1794, 77.1244)
  line L479 (-34.1794, 77.1244) -> (-34.1794, 72.1244)
  line L480 (-34.1794, 72.1244) -> (-29.8493, 69.6244)
  line L481 (-29.8493, 69.6244) -> (-25.5191, 72.1244)
  line L482 (-25.5191, 72.1244) -> (-25.5191, 77.1244)
  line L483 (-25.5191, 77.1244) -> (-29.8493, 79.6244)
  line L484 (-19.189, 79.6244) -> (-23.5191, 77.1244)
  line L485 (-23.5191, 77.1244) -> (-23.5191, 72.1244)
  line L486 (-23.5191, 72.1244) -> (-19.189, 69.6244)
  line L487 (-19.189, 69.6244) -> (-14.8589, 72.1244)
  line L488 (-14.8589, 72.1244) -> (-14.8589, 77.1244)
  line L489 (-14.8589, 77.1244) -> (-19.189, 79.6244)
  line L490 (-8.5287, 79.6244) -> (-12.8589, 77.1244)
  line L491 (-12.8589, 77.1244) -> (-12.8589, 72.1244)
  line L492 (-12.8589, 72.1244) -> (-8.5287, 69.6244)
  line L493 (-8.5287, 69.6244) -> (-4.1986, 72.1244)
  line L494 (-4.1986, 72.1244) -> (-4.1986, 77.1244)
  line L495 (-4.1986, 77.1244) -> (-8.5287, 79.6244)
  line L496 (2.1315, 79.6244) -> (-2.1986, 77.1244)
  line L497 (-2.1986, 77.1244) -> (-2.1986, 72.1244)
  line L498 (-2.1986, 72.1244) -> (2.1315, 69.6244)
  line L499 (2.1315, 69.6244) -> (6.4616, 72.1244)
  line L500 (6.4616, 72.1244) -> (6.4616, 77.1244)
  line L501 (6.4616, 77.1244) -> (2.1315, 79.6244)
  line L502 (12.7918, 79.6244) -> (8.4616, 77.1244)
  line L503 (8.4616, 77.1244) -> (8.4616, 72.1244)
  line L504 (8.4616, 72.1244) -> (12.7918, 69.6244)
  line L505 (12.7918, 69.6244) -> (17.1219, 72.1244)
  line L506 (17.1219, 72.1244) -> (17.1219, 77.1244)
  line L507 (17.1219, 77.1244) -> (12.7918, 79.6244)
  line L508 (23.452, 79.6244) -> (19.1219, 77.1244)
  line L509 (19.1219, 77.1244) -> (19.1219, 72.1244)
  line L510 (19.1219, 72.1244) -> (23.452, 69.6244)
  line L511 (23.452, 69.6244) -> (27.7821, 72.1244)
  line L512 (27.7821, 72.1244) -> (27.7821, 77.1244)
  line L513 (27.7821, 77.1244) -> (23.452, 79.6244)
  line L514 (34.1123, 79.6244) -> (29.7821, 77.1244)
  line L515 (29.7821, 77.1244) -> (29.7821, 72.1244)
  line L516 (29.7821, 72.1244) -> (34.1123, 69.6244)
  line L517 (34.1123, 69.6244) -> (38.4424, 72.1244)
  line L518 (38.4424, 72.1244) -> (38.4424, 77.1244)
  line L519 (38.4424, 77.1244) -> (34.1123, 79.6244)
  line L520 (44.7725, 79.6244) -> (40.4424, 77.1244)
  line L521 (40.4424, 77.1244) -> (40.4424, 72.1244)
  line L522 (40.4424, 72.1244) -> (44.7725, 69.6244)
  line L523 (44.7725, 69.6244) -> (49.1027, 72.1244)
  line L524 (49.1027, 72.1244) -> (49.1027, 77.1244)
  line L525 (49.1027, 77.1244) -> (44.7725, 79.6244)
  line L526 (55.4328, 79.6244) -> (51.1027, 77.1244)
  line L527 (51.1027, 77.1244) -> (51.1027, 72.1244)
  line L528 (51.1027, 72.1244) -> (55.4328, 69.6244)
  line L529 (55.4328, 69.6244) -> (59.7629, 72.1244)
  line L530 (59.7629, 72.1244) -> (59.7629, 77.1244)
  line L531 (59.7629, 77.1244) -> (55.4328, 79.6244)
  line L532 (-56.4999, 88.8564) -> (-60.83, 86.3564)
  line L533 (-60.83, 86.3564) -> (-60.83, 81.3564)
  line L534 (-60.83, 81.3564) -> (-56.4999, 78.8564)
  line L535 (-56.4999, 78.8564) -> (-52.1698, 81.3564)
  line L536 (-52.1698, 81.3564) -> (-52.1698, 86.3564)
  line L537 (-52.1698, 86.3564) -> (-56.4999, 88.8564)
  line L538 (-45.8396, 88.8564) -> (-50.1698, 86.3564)
  line L539 (-50.1698, 86.3564) -> (-50.1698, 81.3564)
  line L540 (-50.1698, 81.3564) -> (-45.8396, 78.8564)
  line L541 (-45.8396, 78.8564) -> (-41.5095, 81.3564)
  line L542 (-41.5095, 81.3564) -> (-41.5095, 86.3564)
  line L543 (-41.5095, 86.3564) -> (-45.8396, 88.8564)
  line L544 (-35.1794, 88.8564) -> (-39.5095, 86.3564)
  line L545 (-39.5095, 86.3564) -> (-39.5095, 81.3564)
  line L546 (-39.5095, 81.3564) -> (-35.1794, 78.8564)
  line L547 (-35.1794, 78.8564) -> (-30.8493, 81.3564)
  line L548 (-30.8493, 81.3564) -> (-30.8493, 86.3564)
  line L549 (-30.8493, 86.3564) -> (-35.1794, 88.8564)
  line L550 (-24.5191, 88.8564) -> (-28.8493, 86.3564)
  line L551 (-28.8493, 86.3564) -> (-28.8493, 81.3564)
  line L552 (-28.8493, 81.3564) -> (-24.5191, 78.8564)
  line L553 (-24.5191, 78.8564) -> (-20.189, 81.3564)
  line L554 (-20.189, 81.3564) -> (-20.189, 86.3564)
  line L555 (-20.189, 86.3564) -> (-24.5191, 88.8564)
  line L556 (-13.8589, 88.8564) -> (-18.189, 86.3564)
  line L557 (-18.189, 86.3564) -> (-18.189, 81.3564)
  line L558 (-18.189, 81.3564) -> (-13.8589, 78.8564)
  line L559 (-13.8589, 78.8564) -> (-9.5287, 81.3564)
  line L560 (-9.5287, 81.3564) -> (-9.5287, 86.3564)
  line L561 (-9.5287, 86.3564) -> (-13.8589, 88.8564)
  line L562 (-3.1986, 88.8564) -> (-7.5287, 86.3564)
  line L563 (-7.5287, 86.3564) -> (-7.5287, 81.3564)
  line L564 (-7.5287, 81.3564) -> (-3.1986, 78.8564)
  line L565 (-3.1986, 78.8564) -> (1.1315, 81.3564)
  line L566 (1.1315, 81.3564) -> (1.1315, 86.3564)
  line L567 (1.1315, 86.3564) -> (-3.1986, 88.8564)
  line L568 (7.4616, 88.8564) -> (3.1315, 86.3564)
  line L569 (3.1315, 86.3564) -> (3.1315, 81.3564)
  line L570 (3.1315, 81.3564) -> (7.4616, 78.8564)
  line L571 (7.4616, 78.8564) -> (11.7918, 81.3564)
  line L572 (11.7918, 81.3564) -> (11.7918, 86.3564)
  line L573 (11.7918, 86.3564) -> (7.4616, 88.8564)
  line L574 (18.1219, 88.8564) -> (13.7918, 86.3564)
  line L575 (13.7918, 86.3564) -> (13.7918, 81.3564)
  line L576 (13.7918, 81.3564) -> (18.1219, 78.8564)
  line L577 (18.1219, 78.8564) -> (22.452, 81.3564)
  line L578 (22.452, 81.3564) -> (22.452, 86.3564)
  line L579 (22.452, 86.3564) -> (18.1219, 88.8564)
  line L580 (28.7821, 88.8564) -> (24.452, 86.3564)
  line L581 (24.452, 86.3564) -> (24.452, 81.3564)
  line L582 (24.452, 81.3564) -> (28.7821, 78.8564)
  line L583 (28.7821, 78.8564) -> (33.1123, 81.3564)
  line L584 (33.1123, 81.3564) -> (33.1123, 86.3564)
  line L585 (33.1123, 86.3564) -> (28.7821, 88.8564)
  line L586 (39.4424, 88.8564) -> (35.1123, 86.3564)
  line L587 (35.1123, 86.3564) -> (35.1123, 81.3564)
  line L588 (35.1123, 81.3564) -> (39.4424, 78.8564)
  line L589 (39.4424, 78.8564) -> (43.7725, 81.3564)
  line L590 (43.7725, 81.3564) -> (43.7725, 86.3564)
  line L591 (43.7725, 86.3564) -> (39.4424, 88.8564)
  line L592 (50.1027, 88.8564) -> (45.7725, 86.3564)
  line L593 (45.7725, 86.3564) -> (45.7725, 81.3564)
  line L594 (45.7725, 81.3564) -> (50.1027, 78.8564)
  line L595 (50.1027, 78.8564) -> (54.4328, 81.3564)
  line L596 (54.4328, 81.3564) -> (54.4328, 86.3564)
  line L597 (54.4328, 86.3564) -> (50.1027, 88.8564)
  line L598 (-51.1698, 98.0885) -> (-55.4999, 95.5885)
  line L599 (-55.4999, 95.5885) -> (-55.4999, 90.5885)
  line L600 (-55.4999, 90.5885) -> (-51.1698, 88.0885)
  line L601 (-51.1698, 88.0885) -> (-46.8396, 90.5885)
  line L602 (-46.8396, 90.5885) -> (-46.8396, 95.5885)
  line L603 (-46.8396, 95.5885) -> (-51.1698, 98.0885)
  line L604 (-40.5095, 98.0885) -> (-44.8396, 95.5885)
  line L605 (-44.8396, 95.5885) -> (-44.8396, 90.5885)
  line L606 (-44.8396, 90.5885) -> (-40.5095, 88.0885)
  line L607 (-40.5095, 88.0885) -> (-36.1794, 90.5885)
  line L608 (-36.1794, 90.5885) -> (-36.1794, 95.5885)
  line L609 (-36.1794, 95.5885) -> (-40.5095, 98.0885)
  line L610 (-29.8493, 98.0885) -> (-34.1794, 95.5885)
  line L611 (-34.1794, 95.5885) -> (-34.1794, 90.5885)
  line L612 (-34.1794, 90.5885) -> (-29.8493, 88.0885)
  line L613 (-29.8493, 88.0885) -> (-25.5191, 90.5885)
  line L614 (-25.5191, 90.5885) -> (-25.5191, 95.5885)
  line L615 (-25.5191, 95.5885) -> (-29.8493, 98.0885)
  line L616 (-19.189, 98.0885) -> (-23.5191, 95.5885)
  line L617 (-23.5191, 95.5885) -> (-23.5191, 90.5885)
  line L618 (-23.5191, 90.5885) -> (-19.189, 88.0885)
  line L619 (-19.189, 88.0885) -> (-14.8589, 90.5885)
  line L620 (-14.8589, 90.5885) -> (-14.8589, 95.5885)
  line L621 (-14.8589, 95.5885) -> (-19.189, 98.0885)
  line L622 (-8.5287, 98.0885) -> (-12.8589, 95.5885)
  line L623 (-12.8589, 95.5885) -> (-12.8589, 90.5885)
  line L624 (-12.8589, 90.5885) -> (-8.5287, 88.0885)
  line L625 (-8.5287, 88.0885) -> (-4.1986, 90.5885)
  line L626 (-4.1986, 90.5885) -> (-4.1986, 95.5885)
  line L627 (-4.1986, 95.5885) -> (-8.5287, 98.0885)
  line L628 (2.1315, 98.0885) -> (-2.1986, 95.5885)
  line L629 (-2.1986, 95.5885) -> (-2.1986, 90.5885)
  line L630 (-2.1986, 90.5885) -> (2.1315, 88.0885)
  line L631 (2.1315, 88.0885) -> (6.4616, 90.5885)
  line L632 (6.4616, 90.5885) -> (6.4616, 95.5885)
  line L633 (6.4616, 95.5885) -> (2.1315, 98.0885)
  line L634 (12.7918, 98.0885) -> (8.4616, 95.5885)
  line L635 (8.4616, 95.5885) -> (8.4616, 90.5885)
  line L636 (8.4616, 90.5885) -> (12.7918, 88.0885)
  line L637 (12.7918, 88.0885) -> (17.1219, 90.5885)
  line L638 (17.1219, 90.5885) -> (17.1219, 95.5885)
  line L639 (17.1219, 95.5885) -> (12.7918, 98.0885)
  line L640 (23.452, 98.0885) -> (19.1219, 95.5885)
  line L641 (19.1219, 95.5885) -> (19.1219, 90.5885)
  line L642 (19.1219, 90.5885) -> (23.452, 88.0885)
  line L643 (23.452, 88.0885) -> (27.7821, 90.5885)
  line L644 (27.7821, 90.5885) -> (27.7821, 95.5885)
  line L645 (27.7821, 95.5885) -> (23.452, 98.0885)
  line L646 (34.1123, 98.0885) -> (29.7821, 95.5885)
  line L647 (29.7821, 95.5885) -> (29.7821, 90.5885)
  line L648 (29.7821, 90.5885) -> (34.1123, 88.0885)
  line L649 (34.1123, 88.0885) -> (38.4424, 90.5885)
  line L650 (38.4424, 90.5885) -> (38.4424, 95.5885)
  line L651 (38.4424, 95.5885) -> (34.1123, 98.0885)
  line L652 (44.7725, 98.0885) -> (40.4424, 95.5885)
  line L653 (40.4424, 95.5885) -> (40.4424, 90.5885)
  line L654 (40.4424, 90.5885) -> (44.7725, 88.0885)
  line L655 (44.7725, 88.0885) -> (49.1027, 90.5885)
  line L656 (49.1027, 90.5885) -> (49.1027, 95.5885)
  line L657 (49.1027, 95.5885) -> (44.7725, 98.0885)
  line L658 (55.4328, 98.0885) -> (51.1027, 95.5885)
  line L659 (51.1027, 95.5885) -> (51.1027, 90.5885)
  line L660 (51.1027, 90.5885) -> (55.4328, 88.0885)
  line L661 (55.4328, 88.0885) -> (59.7629, 90.5885)
  line L662 (59.7629, 90.5885) -> (59.7629, 95.5885)
  line L663 (59.7629, 95.5885) -> (55.4328, 98.0885)
  line L664 (-56.4999, 107.3205) -> (-60.83, 104.8205)
  line L665 (-60.83, 104.8205) -> (-60.83, 99.8205)
  line L666 (-60.83, 99.8205) -> (-56.4999, 97.3205)
  line L667 (-56.4999, 97.3205) -> (-52.1698, 99.8205)
  line L668 (-52.1698, 99.8205) -> (-52.1698, 104.8205)
  line L669 (-52.1698, 104.8205) -> (-56.4999, 107.3205)
  line L670 (-45.8396, 107.3205) -> (-50.1698, 104.8205)
  line L671 (-50.1698, 104.8205) -> (-50.1698, 99.8205)
  line L672 (-50.1698, 99.8205) -> (-45.8396, 97.3205)
  line L673 (-45.8396, 97.3205) -> (-41.5095, 99.8205)
  line L674 (-41.5095, 99.8205) -> (-41.5095, 104.8205)
  line L675 (-41.5095, 104.8205) -> (-45.8396, 107.3205)
  line L676 (-35.1794, 107.3205) -> (-39.5095, 104.8205)
  line L677 (-39.5095, 104.8205) -> (-39.5095, 99.8205)
  line L678 (-39.5095, 99.8205) -> (-35.1794, 97.3205)
  line L679 (-35.1794, 97.3205) -> (-30.8493, 99.8205)
  line L680 (-30.8493, 99.8205) -> (-30.8493, 104.8205)
  line L681 (-30.8493, 104.8205) -> (-35.1794, 107.3205)
  line L682 (-24.5191, 107.3205) -> (-28.8493, 104.8205)
  line L683 (-28.8493, 104.8205) -> (-28.8493, 99.8205)
  line L684 (-28.8493, 99.8205) -> (-24.5191, 97.3205)
  line L685 (-24.5191, 97.3205) -> (-20.189, 99.8205)
  line L686 (-20.189, 99.8205) -> (-20.189, 104.8205)
  line L687 (-20.189, 104.8205) -> (-24.5191, 107.3205)
  line L688 (-13.8589, 107.3205) -> (-18.189, 104.8205)
  line L689 (-18.189, 104.8205) -> (-18.189, 99.8205)
  line L690 (-18.189, 99.8205) -> (-13.8589, 97.3205)
  line L691 (-13.8589, 97.3205) -> (-9.5287, 99.8205)
  line L692 (-9.5287, 99.8205) -> (-9.5287, 104.8205)
  line L693 (-9.5287, 104.8205) -> (-13.8589, 107.3205)
  line L694 (-3.1986, 107.3205) -> (-7.5287, 104.8205)
  line L695 (-7.5287, 104.8205) -> (-7.5287, 99.8205)
  line L696 (-7.5287, 99.8205) -> (-3.1986, 97.3205)
  line L697 (-3.1986, 97.3205) -> (1.1315, 99.8205)
  line L698 (1.1315, 99.8205) -> (1.1315, 104.8205)
  line L699 (1.1315, 104.8205) -> (-3.1986, 107.3205)
  line L700 (7.4616, 107.3205) -> (3.1315, 104.8205)
  line L701 (3.1315, 104.8205) -> (3.1315, 99.8205)
  line L702 (3.1315, 99.8205) -> (7.4616, 97.3205)
  line L703 (7.4616, 97.3205) -> (11.7918, 99.8205)
  line L704 (11.7918, 99.8205) -> (11.7918, 104.8205)
  line L705 (11.7918, 104.8205) -> (7.4616, 107.3205)
  line L706 (18.1219, 107.3205) -> (13.7918, 104.8205)
  line L707 (13.7918, 104.8205) -> (13.7918, 99.8205)
  line L708 (13.7918, 99.8205) -> (18.1219, 97.3205)
  line L709 (18.1219, 97.3205) -> (22.452, 99.8205)
  line L710 (22.452, 99.8205) -> (22.452, 104.8205)
  line L711 (22.452, 104.8205) -> (18.1219, 107.3205)
  line L712 (28.7821, 107.3205) -> (24.452, 104.8205)
  line L713 (24.452, 104.8205) -> (24.452, 99.8205)
  line L714 (24.452, 99.8205) -> (28.7821, 97.3205)
  line L715 (28.7821, 97.3205) -> (33.1123, 99.8205)
  line L716 (33.1123, 99.8205) -> (33.1123, 104.8205)
  line L717 (33.1123, 104.8205) -> (28.7821, 107.3205)
  line L718 (39.4424, 107.3205) -> (35.1123, 104.8205)
  line L719 (35.1123, 104.8205) -> (35.1123, 99.8205)
  line L720 (35.1123, 99.8205) -> (39.4424, 97.3205)
  line L721 (39.4424, 97.3205) -> (43.7725, 99.8205)
  line L722 (43.7725, 99.8205) -> (43.7725, 104.8205)
  line L723 (43.7725, 104.8205) -> (39.4424, 107.3205)
  line L724 (50.1027, 107.3205) -> (45.7725, 104.8205)
  line L725 (45.7725, 104.8205) -> (45.7725, 99.8205)
  line L726 (45.7725, 99.8205) -> (50.1027, 97.3205)
  line L727 (50.1027, 97.3205) -> (54.4328, 99.8205)
  line L728 (54.4328, 99.8205) -> (54.4328, 104.8205)
  line L729 (54.4328, 104.8205) -> (50.1027, 107.3205)
  line L730 (-51.1698, 116.5526) -> (-55.4999, 114.0526)
  line L731 (-55.4999, 114.0526) -> (-55.4999, 109.0526)
  line L732 (-55.4999, 109.0526) -> (-51.1698, 106.5526)
  line L733 (-51.1698, 106.5526) -> (-46.8396, 109.0526)
  line L734 (-46.8396, 109.0526) -> (-46.8396, 114.0526)
  line L735 (-46.8396, 114.0526) -> (-51.1698, 116.5526)
  line L736 (-40.5095, 116.5526) -> (-44.8396, 114.0526)
  line L737 (-44.8396, 114.0526) -> (-44.8396, 109.0526)
  line L738 (-44.8396, 109.0526) -> (-40.5095, 106.5526)
  line L739 (-40.5095, 106.5526) -> (-36.1794, 109.0526)
  line L740 (-36.1794, 109.0526) -> (-36.1794, 114.0526)
  line L741 (-36.1794, 114.0526) -> (-40.5095, 116.5526)
  line L742 (-29.8493, 116.5526) -> (-34.1794, 114.0526)
  line L743 (-34.1794, 114.0526) -> (-34.1794, 109.0526)
  line L744 (-34.1794, 109.0526) -> (-29.8493, 106.5526)
  line L745 (-29.8493, 106.5526) -> (-25.5191, 109.0526)
  line L746 (-25.5191, 109.0526) -> (-25.5191, 114.0526)
  line L747 (-25.5191, 114.0526) -> (-29.8493, 116.5526)
  line L748 (-19.189, 116.5526) -> (-23.5191, 114.0526)
  line L749 (-23.5191, 114.0526) -> (-23.5191, 109.0526)
  line L750 (-23.5191, 109.0526) -> (-19.189, 106.5526)
  line L751 (-19.189, 106.5526) -> (-14.8589, 109.0526)
  line L752 (-14.8589, 109.0526) -> (-14.8589, 114.0526)
  line L753 (-14.8589, 114.0526) -> (-19.189, 116.5526)
  line L754 (-8.5287, 116.5526) -> (-12.8589, 114.0526)
  line L755 (-12.8589, 114.0526) -> (-12.8589, 109.0526)
  line L756 (-12.8589, 109.0526) -> (-8.5287, 106.5526)
  line L757 (-8.5287, 106.5526) -> (-4.1986, 109.0526)
  line L758 (-4.1986, 109.0526) -> (-4.1986, 114.0526)
  line L759 (-4.1986, 114.0526) -> (-8.5287, 116.5526)
  line L760 (2.1315, 116.5526) -> (-2.1986, 114.0526)
  line L761 (-2.1986, 114.0526) -> (-2.1986, 109.0526)
  line L762 (-2.1986, 109.0526) -> (2.1315, 106.5526)
  line L763 (2.1315, 106.5526) -> (6.4616, 109.0526)
  line L764 (6.4616, 109.0526) -> (6.4616, 114.0526)
  line L765 (6.4616, 114.0526) -> (2.1315, 116.5526)
  line L766 (12.7918, 116.5526) -> (8.4616, 114.0526)
  line L767 (8.4616, 114.0526) -> (8.4616, 109.0526)
  line L768 (8.4616, 109.0526) -> (12.7918, 106.5526)
  line L769 (12.7918, 106.5526) -> (17.1219, 109.0526)
  line L770 (17.1219, 109.0526) -> (17.1219, 114.0526)
  line L771 (17.1219, 114.0526) -> (12.7918, 116.5526)
  line L772 (23.452, 116.5526) -> (19.1219, 114.0526)
  line L773 (19.1219, 114.0526) -> (19.1219, 109.0526)
  line L774 (19.1219, 109.0526) -> (23.452, 106.5526)
  line L775 (23.452, 106.5526) -> (27.7821, 109.0526)
  line L776 (27.7821, 109.0526) -> (27.7821, 114.0526)
  line L777 (27.7821, 114.0526) -> (23.452, 116.5526)
  line L778 (34.1123, 116.5526) -> (29.7821, 114.0526)
  line L779 (29.7821, 114.0526) -> (29.7821, 109.0526)
  line L780 (29.7821, 109.0526) -> (34.1123, 106.5526)
  line L781 (34.1123, 106.5526) -> (38.4424, 109.0526)
  line L782 (38.4424, 109.0526) -> (38.4424, 114.0526)
  line L783 (38.4424, 114.0526) -> (34.1123, 116.5526)
  line L784 (44.7725, 116.5526) -> (40.4424, 114.0526)
  line L785 (40.4424, 114.0526) -> (40.4424, 109.0526)
  line L786 (40.4424, 109.0526) -> (44.7725, 106.5526)
  line L787 (44.7725, 106.5526) -> (49.1027, 109.0526)
  line L788 (49.1027, 109.0526) -> (49.1027, 114.0526)
  line L789 (49.1027, 114.0526) -> (44.7725, 116.5526)
  line L790 (55.4328, 116.5526) -> (51.1027, 114.0526)
  line L791 (51.1027, 114.0526) -> (51.1027, 109.0526)
  line L792 (51.1027, 109.0526) -> (55.4328, 106.5526)
  line L793 (55.4328, 106.5526) -> (59.7629, 109.0526)
  line L794 (59.7629, 109.0526) -> (59.7629, 114.0526)
  line L795 (59.7629, 114.0526) -> (55.4328, 116.5526)
  line L796 (-56.4999, 125.7846) -> (-60.83, 123.2846)
  line L797 (-60.83, 123.2846) -> (-60.83, 118.2846)
  line L798 (-60.83, 118.2846) -> (-56.4999, 115.7846)
  line L799 (-56.4999, 115.7846) -> (-52.1698, 118.2846)
  line L800 (-52.1698, 118.2846) -> (-52.1698, 123.2846)
  line L801 (-52.1698, 123.2846) -> (-56.4999, 125.7846)
  line L802 (-45.8396, 125.7846) -> (-50.1698, 123.2846)
  line L803 (-50.1698, 123.2846) -> (-50.1698, 118.2846)
  line L804 (-50.1698, 118.2846) -> (-45.8396, 115.7846)
  line L805 (-45.8396, 115.7846) -> (-41.5095, 118.2846)
  line L806 (-41.5095, 118.2846) -> (-41.5095, 123.2846)
  line L807 (-41.5095, 123.2846) -> (-45.8396, 125.7846)
  line L808 (-35.1794, 125.7846) -> (-39.5095, 123.2846)
  line L809 (-39.5095, 123.2846) -> (-39.5095, 118.2846)
  line L810 (-39.5095, 118.2846) -> (-35.1794, 115.7846)
  line L811 (-35.1794, 115.7846) -> (-30.8493, 118.2846)
  line L812 (-30.8493, 118.2846) -> (-30.8493, 123.2846)
  line L813 (-30.8493, 123.2846) -> (-35.1794, 125.7846)
  line L814 (-24.5191, 125.7846) -> (-28.8493, 123.2846)
  line L815 (-28.8493, 123.2846) -> (-28.8493, 118.2846)
  line L816 (-28.8493, 118.2846) -> (-24.5191, 115.7846)
  line L817 (-24.5191, 115.7846) -> (-20.189, 118.2846)
  line L818 (-20.189, 118.2846) -> (-20.189, 123.2846)
  line L819 (-20.189, 123.2846) -> (-24.5191, 125.7846)
  line L820 (-13.8589, 125.7846) -> (-18.189, 123.2846)
  line L821 (-18.189, 123.2846) -> (-18.189, 118.2846)
  line L822 (-18.189, 118.2846) -> (-13.8589, 115.7846)
  line L823 (-13.8589, 115.7846) -> (-9.5287, 118.2846)
  line L824 (-9.5287, 118.2846) -> (-9.5287, 123.2846)
  line L825 (-9.5287, 123.2846) -> (-13.8589, 125.7846)
  line L826 (-3.1986, 125.7846) -> (-7.5287, 123.2846)
  line L827 (-7.5287, 123.2846) -> (-7.5287, 118.2846)
  line L828 (-7.5287, 118.2846) -> (-3.1986, 115.7846)
  line L829 (-3.1986, 115.7846) -> (1.1315, 118.2846)
  line L830 (1.1315, 118.2846) -> (1.1315, 123.2846)
  line L831 (1.1315, 123.2846) -> (-3.1986, 125.7846)
  line L832 (7.4616, 125.7846) -> (3.1315, 123.2846)
  line L833 (3.1315, 123.2846) -> (3.1315, 118.2846)